connector_dual_magnet (Autodesk Fusion 360 design; units mm, degrees)
Autodesk Fusion 360 part; units mm, degrees
note: some values were not read from the file. Set by a fixed rule: which sketch regions a step uses.
sketch "Sketch1" plane through (0, 0, 0) normal (0, 1, 0) x (1, 0, 0)
  line L0 (0, 0) -> (-21, 0) construction
  line L1 (-10, 0) -> (-18, 0)
  arc A0 (-10, 0) -> (-18, 0) centre (-14, 0) ccw
  arc A1 (-18, 0) -> (-10, 0) centre (-14, 0) ccw
  line L2 (0, 0) -> (-8, 0)
  arc A2 (0, 0) -> (-8, 0) centre (-4, 0) ccw
  arc A3 (-8, 0) -> (0, 0) centre (-4, 0) ccw
  circle A4 centre (-21, 0) radius 2
  line L3 (-4, 0) -> (-14, 0) construction
  line L4 (-9, 2.7) -> (-9, -2.7) construction
  circle A5 centre (-9, -2.7) radius 1
  circle A6 centre (-9, 2.7) radius 1
  line L5 (-4, 0) -> (-4, -5.4) construction
  line L6 (-4, 0) -> (-4, 5.4) construction
  line L7 (-21, 0) -> (-21, -3) construction
  line L8 (-21, 0) -> (-21, 3) construction
  line L9 (-14, 0) -> (-14, 4.75) construction
  circle A7 centre (-14, 0) radius 4.75
  line L10 (-9, -1.7) -> (-9, -3.7)
  line L11 (-9, 3.7) -> (-9, 1.7)
  circle A8 centre (-9, 2.7) radius 1.75
  circle A9 centre (-9, -2.7) radius 1.75
  circle A10 centre (-4, 0) radius 4.75
  line L12 (-4.2898, 4.7412) -> (-9.1068, 4.4467)
  line L13 (-8.8932, 4.4467) -> (-13.7102, 4.7412)
  line L14 (-15.3571, 4.552) -> (-21.7857, 2.6354)
  line L15 (-21.7857, -2.6354) -> (-15.3571, -4.552)
  line L16 (-13.7102, -4.7412) -> (-8.8932, -4.4467)
  line L17 (-9.1068, -4.4467) -> (-4.2898, -4.7412)
  circle A11 centre (-21, 0) radius 2.75
  dimension "d4" = 8
  dimension "d5" = 8
  dimension "d22" = 4
  dimension "d27" = 10
  dimension "d28" = 7
  dimension "d29" = 2
  dimension "d30" = 2
  dimension "d31" = 5.4
  dimension "d41" = 3.5
  dimension "d42" = 3.5
  dimension "d43" = 9.5
  dimension "d44" = 9.5
  dimension "d45" = 5.5
  constraint coincident L0 A2.centre
  constraint coincident L0 A0.centre
  constraint coincident L0 L1.start
  constraint coincident L0 L1.end
  constraint coincident A0.centre A1.centre
  constraint coincident L0 L2.start
  constraint coincident L0 L2.end
  constraint coincident A2.centre A3.centre
  constraint coincident L0 A4.centre
  constraint coincident L0.start L2.start
  constraint horizontal L0
  constraint coincident L0.end A4.centre
  constraint vertical L4
  constraint midpoint L3 L4
  constraint coincident L4.end A5.centre
  constraint coincident L4.start A6.centre
  constraint vertical L5
  constraint vertical L6
  constraint vertical L7
  constraint vertical L8
  constraint vertical L9
  constraint concentric A1 A7
  constraint coincident L9.end A7
  constraint coincident A5 L10.start
  constraint coincident L4 L10.start
  constraint coincident A5 L10.end
  constraint parallel L4 L10
  constraint coincident A6 L11.start
  constraint coincident A6 L11.end
  constraint coincident L4 L11.end
  constraint parallel L4 L11
  constraint concentric A5 A9
  constraint concentric A3 A10
  constraint tangent A10 L17
  constraint tangent A9 L17
  constraint tangent A7 L16
  constraint tangent A9 L16
  constraint tangent A7 L15
  constraint tangent A7 L14
  constraint tangent A7 L13
  constraint tangent A8 L13
  constraint tangent A8 L12
  constraint tangent A10 L12
  constraint coincident A10 L12.start
  constraint coincident A10 L17.end
  constraint coincident A9 L17.start
  constraint coincident A9 L16.end
  constraint coincident A7 L16.start
  constraint coincident A7 L15.end
  constraint coincident A7 L14.start
  constraint coincident A7 L13.end
  constraint coincident A8 L13.start
  constraint coincident A8 L12.end
  constraint concentric A4 A11
  constraint tangent L15 A11
  constraint tangent L14 A11
  constraint coincident L14.end A11
  constraint coincident L15.start A11
  measures "d4" diameter of A2
  measures "d5" diameter of A0
  measures "d22" diameter of A4
  measures "d27" distance of A0.centre A2.centre
  measures "d28" distance of A0.centre L0.end
  measures "d29" diameter of A5
  measures "d30" diameter of A6
  measures "d31" distance of L4.start L4.end
  measures "d41" diameter of A9
  measures "d42" diameter of A8
  measures "d43" diameter of A7
  measures "d44" diameter of A10
  measures "d45" diameter of A11
extrude "Extrude3" add sketch "Sketch1" along normal blind 3 contours A0 A1 A7 A8 A9 | A0 A1 A7 A8 A9 A11 | A0 A6 A7 A8 | A1 A5 A7 A9 | A7 A8 A9 A10 | A6 A7 A8 A10 | A5 A7 A9 A10 | A6 A7 A8 A10 | A7 A8 L12 L13 | A7 A9 L16 L17 | A5 A7 A9 A10 | A6 A7 L11 | A6 A7 | A2 A6 A8 A10 | A2 A3 A8 A9 A10 | A5 A7 | A5 A7 L10 | A3 A5 A9 A10 | A6 L11 A10 | A6 A10 | A5 L10 A10 | A5 A10 | A7 L14 A11 | A8 A10 L12 L13 | A7 L15 A11 | A9 A10 L16 L17 | A2 A3 A8 A9 A10 | A7 A11 | A7 A11
revolve "Revolve3" add sketch "Sketch1" angle 360 about axis through (-9, 0, 1.7) along (0, 0, 1) contours A6 L11 A10 | A6 A10 | A5 L10 A10 | A5 A10
sketch "Sketch2" plane through (0, 3, 0) normal (0, 1, 0) x (-1, 0, 0)
  circle A0 centre (14, 0) radius 4
  circle A1 centre (9, -2.7) radius 1
  circle A2 centre (9, -2.7) radius 1
  circle A3 centre (9, 2.7) radius 1
  circle A4 centre (9, 2.7) radius 1
  line L0 (9, 3.7) -> (9, 1.7)
  line L1 (9, -1.7) -> (9, -3.7)
  circle A5 centre (4, 0) radius 4
  arc A6 (8.8932, -4.4467) -> (9.1068, -4.4467) centre (9, -2.7) ccw
  line L2 (9.1068, -4.4467) -> (9, -4.4533)
  line L3 (9, -4.4533) -> (13.7102, -4.7412)
  arc A7 (13.7102, -4.7412) -> (15.3571, -4.552) centre (14, 0) ccw
  line L4 (13.7102, 4.7412) -> (9, 4.4533)
  line L5 (9, 4.4533) -> (9.1068, 4.4467)
  arc A8 (9.1068, 4.4467) -> (8.8932, 4.4467) centre (9, 2.7) ccw
  line L6 (8.8932, 4.4467) -> (9, 4.4533)
  line L7 (9, 4.4533) -> (4.2898, 4.7412)
  arc A9 (4.2898, 4.7412) -> (4.2898, -4.7412) centre (4, 0) ccw
  line L8 (4.2898, -4.7412) -> (9, -4.4533)
  line L9 (9, -4.4533) -> (8.8932, -4.4467)
  line L10 (21.7857, 2.6354) -> (15.3571, 4.552)
  arc A10 (15.3571, 4.552) -> (13.7102, 4.7412) centre (14, 0) ccw
  arc A11 (21.7857, -2.6354) -> (21.7857, 2.6354) centre (21, 0) ccw
  circle A12 centre (21, 0) radius 2
  line L11 (15.3571, -4.552) -> (21.7857, -2.6354)
  dimension "d37" = 2
  dimension "d38" = 2
  constraint concentric A1 A2
  constraint concentric A3 A4
  constraint coincident A4 L0.start
  constraint coincident A4 L0.end
  constraint vertical L0
  constraint coincident A2 L1.start
  constraint coincident A1 L1.end
  constraint parallel L0 L1
  constraint midpoint A1.centre L1
  constraint midpoint A3.centre L0
  measures "d37" diameter of A1
  measures "d38" diameter of A3
revolve "Revolve4" cut sketch "Sketch2" angle 360 about axis through (-9, 3, -1.7) along (0, 0, -1) contours A1 A2 L1 | A3 A4 L0 picked at (9.3244, -3.0299) picked at (9.3596, 2.9418)
move_face "OffsetFaces2" offset -0.1 2 faces at (-8.0519, 2.7636, -2.9128) (-8.0519, 2.7636, 2.4872)
equation "d2 = 5 mm"
equation "d5 = d4"
equation "d6 = d4 / 2 + d2 / 2 + 1 mm"
equation "d27 = d5 + 2 mm"
equation "d28 = d5 / 2 + d22 / 2 + 1 mm"
equation "d41 = d29 + 1.5 mm"
equation "d42 = d41"
equation "d43 = d5 + 1.5 mm"
equation "d44 = d43"
equation "d45 = d22 + 1.5 mm"
